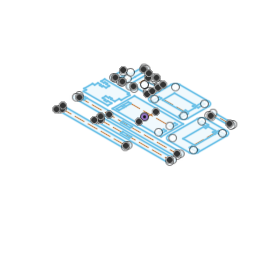
laser cut parts v7 (Autodesk Fusion 360 design; units mm, degrees)
Autodesk Fusion 360 part; units mm, degrees
note: some values were not read from the file. Set by a fixed rule: which sketch regions a step uses.
sketch "Sketch1" plane through (0, 0, 0) normal (0, 0, 1) x (1, 0, 0)
  line L0 (-61.9661, -10.0098) -> (-33.3218, -10.0098)
  line L1 (-33.3218, 14.9902) -> (-61.9661, 14.9902)
  line L2 (-33.3218, 13.3981) -> (-30.7818, 13.3981)
  line L3 (-30.7818, 13.3981) -> (-30.7818, 3.3981)
  line L4 (-30.7818, 3.3981) -> (-33.3218, 3.3981)
  line L5 (-61.9661, 3.271) -> (-64.5061, 3.271)
  line L6 (-64.5061, 3.271) -> (-64.5061, -6.729)
  line L7 (-64.5061, -6.729) -> (-61.9661, -6.729)
  line L8 (-58.6214, 11.9525) -> (-55.9714, 11.9525)
  line L9 (-55.9714, 5.9525) -> (-58.6214, 5.9525)
  line L10 (-58.6214, 10.8025) -> (-61.9661, 10.8025)
  line L11 (-58.6214, 7.1025) -> (-61.9661, 7.1025)
  line L12 (-58.6214, 5.9525) -> (-58.6214, 7.1025)
  line L13 (-58.6214, 10.8025) -> (-58.6214, 11.9525)
  line L14 (-61.9661, 14.9902) -> (-61.9661, 10.8025)
  line L15 (-61.9661, 7.1025) -> (-61.9661, 3.271)
  line L16 (-61.9661, -6.729) -> (-61.9661, -10.0098)
  line L17 (-33.3218, 13.3981) -> (-33.3218, 14.9902)
  line L18 (-55.9714, 10.8025) -> (-52.3522, 10.8025)
  line L19 (-55.9714, 7.1025) -> (-52.3522, 7.1025)
  line L20 (-52.3522, 7.1025) -> (-52.3522, 10.8025)
  line L21 (-55.9714, 11.9525) -> (-55.9714, 10.8025)
  line L22 (-55.9714, 7.1025) -> (-55.9714, 5.9525)
  line L23 (-40.6135, -1.7451) -> (-43.9582, -1.7451)
  line L24 (-40.6135, -1.7451) -> (-40.6135, -0.5951)
  line L25 (-40.6135, -0.5951) -> (-37.9635, -0.5951)
  line L26 (-37.9635, -0.5951) -> (-37.9635, -1.7451)
  line L27 (-37.9635, -5.4451) -> (-37.9635, -6.5951)
  line L28 (-37.9635, -6.5951) -> (-40.6135, -6.5951)
  line L29 (-40.6135, -6.5951) -> (-40.6135, -5.4451)
  line L30 (-40.6135, -5.4451) -> (-43.9582, -5.4451)
  line L31 (-43.9582, -1.7451) -> (-43.9582, -5.4451)
  line L32 (-37.9635, -1.7451) -> (-33.3218, -1.7451)
  line L33 (-37.9635, -5.4451) -> (-33.3218, -5.4451)
  line L34 (-33.3218, -10.0098) -> (-33.3218, -5.4451)
  line L35 (-33.3218, -1.7451) -> (-33.3218, 3.3981)
  dimension "d35" = 10
  dimension "d36" = 2.54
  dimension "d37" = 2.54
  dimension "d39" = 6
  dimension "d40" = 2.65
  dimension "d43" = 6
  dimension "d44" = 2.65
  dimension "d113" = 28.6443
  dimension "d114" = 10
  constraint horizontal L0
  constraint vertical L34
  constraint horizontal L1
  constraint vertical L14
  constraint horizontal L2
  constraint vertical L3
  constraint horizontal L4
  constraint coincident L2.start L34
  constraint horizontal L5
  constraint vertical L6
  constraint horizontal L7
  constraint coincident L5.start L14
  constraint horizontal L8
  constraint vertical L21
  constraint horizontal L9
  constraint vertical L12
  constraint perpendicular L10 L14
  constraint coincident L11.end L14
  constraint perpendicular L11 L14
  constraint collinear L12 L13
  constraint collinear L14 L15
  constraint collinear L15 L16
  constraint collinear L17 L34
  constraint perpendicular L18 L21
  constraint coincident L19.start L21
  constraint perpendicular L19 L21
  constraint perpendicular L18 L20
  constraint collinear L21 L22
  constraint horizontal L25
  constraint vertical L26
  constraint horizontal L28
  constraint vertical L29
  constraint collinear L24 L29
  constraint coincident L27.start L26
  constraint collinear L26 L27
  constraint perpendicular L30 L31
  constraint coincident L32.end L34
  constraint perpendicular L32 L34
  constraint perpendicular L33 L34
  constraint collinear L34 L35
  measures "d35" distance of L2.end L3.end
  measures "d36" distance of L2.start L2.end
  measures "d37" distance of L5.start L5.end
  measures "d39" distance of L8.start L9.end
  measures "d40" distance of L8.start L8.end
  measures "d43" distance of L24.end L28.end
  measures "d44" distance of L24.end L25.end
  measures "d113" distance of L1.start L1.end
  measures "d114" distance of L5.end L6.end
sketch "Sketch2" plane through (0, 0, 0) normal (0, 0, 1) x (1, 0, 0)
  line L0 (-27.3063, 15.4747) -> (30.0656, 15.4747)
  line L1 (30.0656, 15.4747) -> (30.0656, -10.5253)
  line L2 (30.0656, -10.5253) -> (-27.3063, -10.5253)
  line L3 (-27.3063, -10.5253) -> (-27.3063, 15.4747)
  line L4 (-21.7678, 5.5369) -> (24.2322, 5.5369) construction
  line L5 (-21.7678, 5.5369) -> (-24.6678, 5.5369)
  line L6 (-24.6678, 5.5369) -> (-24.6678, -0.4631)
  line L7 (-24.6678, -0.4631) -> (-21.7678, -0.4631)
  line L8 (-21.7678, -0.4631) -> (-21.7678, 5.5369)
  line L9 (-21.7678, -2.4631) -> (-24.6678, -2.4631)
  line L10 (-24.6678, -2.4631) -> (-24.6678, -8.4631)
  line L11 (-24.6678, -8.4631) -> (-21.7678, -8.4631)
  line L12 (-21.7678, -8.4631) -> (-21.7678, -2.4631)
  line L13 (24.0392, 11.4747) -> (24.0392, 5.4747)
  line L14 (26.9392, 11.4747) -> (24.0392, 11.4747)
  line L15 (26.9392, 5.4747) -> (26.9392, 11.4747)
  line L16 (24.0392, 5.4747) -> (26.9392, 5.4747)
  line L17 (26.9392, -1.5253) -> (24.0392, -1.5253)
  line L18 (24.0392, -7.5253) -> (26.9392, -7.5253)
  line L19 (26.9392, -7.5253) -> (26.9392, -1.5253)
  line L20 (24.0392, -1.5253) -> (24.0392, -7.5253)
  line L21 (1.5442, 11.8441) -> (1.5442, -8.1559) construction
  circle A0 centre (1.5442, 11.8441) radius 0.85
  circle A1 centre (1.5442, -8.1559) radius 0.8502
  line L22 (-49.0766, 46.3412) -> (-49.0766, 47.8412) construction
  circle A2 centre (-49.0766, 47.8412) radius 1.5
  line L23 (-49.0766, 46.3412) -> (-49.0766, 51.2139) construction
  line L24 (-49.0766, 51.2139) -> (-50.2257, 51.2139)
  line L25 (-51.7257, 49.7139) -> (-51.7257, 37.2072)
  line L26 (-49.0766, 51.2139) -> (-49.0766, 46.3412) construction
  line L27 (-46.3309, 35.2072) -> (-46.3309, 49.7139)
  line L28 (-47.8309, 51.2139) -> (-49.0766, 51.2139)
  line L29 (-46.3309, 35.2072) -> (-46.3309, 21.8412)
  line L30 (-48.3309, 19.8412) -> (-50.3309, 19.8412)
  line L31 (-52.3309, 21.8412) -> (-52.3309, 28.5115)
  line L32 (-64.4221, -95.7993) -> (-64.4221, -95.7993)
  line L33 (-54.3309, 35.2072) -> (-53.7257, 35.2072)
  line L34 (-54.3309, 35.2072) -> (-58.3309, 35.2072)
  line L35 (-60.3309, 33.2072) -> (-60.3309, 21.8412)
  line L36 (-54.3309, 28.5115) -> (-54.3309, 21.8412)
  line L37 (-56.3309, 19.8412) -> (-58.3309, 19.8412)
  line L38 (-49.0766, 28.8412) -> (-49.0766, 23.0481) construction
  circle A3 centre (-49.0766, 23.0481) radius 1.5
  circle A4 centre (-57.3309, 23.0481) radius 1.5
  arc A5 (-60.3309, 21.8412) -> (-58.3309, 19.8412) centre (-58.3309, 21.8412) ccw
  arc A6 (-56.3309, 19.8412) -> (-54.3309, 21.8412) centre (-56.3309, 21.8412) ccw
  arc A7 (-58.3309, 35.2072) -> (-60.3309, 33.2072) centre (-58.3309, 33.2072) ccw
  arc A8 (-52.3309, 21.8412) -> (-50.3309, 19.8412) centre (-50.3309, 21.8412) ccw
  arc A9 (-48.3309, 19.8412) -> (-46.3309, 21.8412) centre (-48.3309, 21.8412) ccw
  arc A10 (-53.7257, 35.2072) -> (-51.7257, 37.2072) centre (-53.7257, 37.2072) ccw
  arc A11 (-50.2257, 51.2139) -> (-51.7257, 49.7139) centre (-50.2257, 49.7139) ccw
  arc A12 (-46.3309, 49.7139) -> (-47.8309, 51.2139) centre (-47.8309, 49.7139) ccw
  line L39 (-37.6449, 41.9803) -> (-37.6449, 24.6803) construction
  circle A13 centre (-37.6449, 41.9803) radius 1.5
  circle A14 centre (-37.6449, 24.6803) radius 1.5
  line L40 (-39.9332, 46.9834) -> (-34.8949, 46.9834)
  line L41 (-34.8949, 20.5727) -> (-39.9332, 20.5727)
  line L42 (-41.9332, 22.5727) -> (-41.9332, 44.9834)
  line L43 (-37.6449, 41.9803) -> (-32.8949, 41.9803) construction
  line L44 (-21.7527, 26.8103) -> (-21.7527, 28.8103)
  line L45 (-23.7527, 30.8103) -> (-32.8949, 30.8103)
  line L46 (-32.8949, 32.8103) -> (-32.8949, 32.9834) construction
  line L47 (-32.8949, 37.8103) -> (-23.8949, 37.8103)
  line L48 (-21.8949, 39.8103) -> (-21.8949, 41.8103)
  line L49 (-23.8949, 43.8103) -> (-32.8949, 43.8103)
  line L50 (-32.8949, 44.9834) -> (-32.8949, 43.8103)
  line L51 (-32.8949, 37.8103) -> (-32.8949, 30.8103)
  line L52 (-32.8949, 24.8103) -> (-32.8949, 22.5727)
  line L53 (-32.8949, 24.8103) -> (-23.7527, 24.8103)
  circle A15 centre (-24.5988, 40.8103) radius 1.5
  circle A16 centre (-24.5988, 27.5507) radius 1.5
  line L54 (-49.0766, 23.0481) -> (-57.3309, 23.0481) construction
  line L55 (-32.8949, 43.8103) -> (-30.3549, 43.8103) construction
  arc A17 (-39.9332, 46.9834) -> (-41.9332, 44.9834) centre (-39.9332, 44.9834) ccw
  arc A18 (-32.8949, 44.9834) -> (-34.8949, 46.9834) centre (-34.8949, 44.9834) ccw
  arc A19 (-41.9332, 22.5727) -> (-39.9332, 20.5727) centre (-39.9332, 22.5727) ccw
  arc A20 (-34.8949, 20.5727) -> (-32.8949, 22.5727) centre (-34.8949, 22.5727) ccw
  arc A21 (-23.7527, 24.8103) -> (-21.7527, 26.8103) centre (-23.7527, 26.8103) ccw
  arc A22 (-21.7527, 28.8103) -> (-23.7527, 30.8103) centre (-23.7527, 28.8103) ccw
  arc A23 (-23.8949, 37.8103) -> (-21.8949, 39.8103) centre (-23.8949, 39.8103) ccw
  arc A24 (-21.8949, 41.8103) -> (-23.8949, 43.8103) centre (-23.8949, 41.8103) ccw
  line L56 (-53.3309, 29.5115) -> (-54.3309, 29.5115)
  line L57 (-54.3309, 29.5115) -> (-54.3309, 28.5115)
  line L58 (-52.3309, 28.5115) -> (-52.3309, 29.5046)
  line L59 (-52.3309, 29.5046) -> (-53.3309, 29.5115)
  line L60 (17.4575, 27.8424) -> (-6.5425, 27.8424)
  line L61 (-6.5425, 27.8424) -> (-6.5425, 41.8424)
  line L62 (-6.5425, 41.8424) -> (17.4575, 41.8424)
  line L63 (27.0896, 48.5722) -> (27.0896, 24.0668)
  line L64 (22.0896, 19.0668) -> (-12.121, 19.0668)
  line L65 (-17.121, 24.0668) -> (-17.121, 48.5722)
  line L66 (-12.121, 53.5722) -> (22.0896, 53.5722)
  line L67 (19.389, 28.8858) -> (-8.997, 28.8858) construction
  line L68 (-8.997, 28.8858) -> (-11.897, 28.8858)
  line L69 (-11.897, 28.8858) -> (-11.897, 21.2858)
  line L70 (-11.897, 21.2858) -> (-8.997, 21.2858)
  line L71 (-8.997, 21.2858) -> (-8.997, 28.8858)
  line L72 (19.389, 28.8858) -> (19.389, 21.2858)
  line L73 (22.289, 28.8858) -> (19.389, 28.8858)
  line L74 (19.389, 21.2858) -> (22.289, 21.2858)
  line L75 (22.289, 21.2858) -> (22.289, 28.8858)
  line L76 (17.4575, 30.8424) -> (20.5266, 30.8424)
  line L77 (20.5266, 30.8424) -> (20.5266, 39.3145)
  line L78 (20.5266, 39.3145) -> (17.4575, 39.3145)
  line L79 (17.4575, 41.8424) -> (17.4575, 39.3145)
  line L80 (17.4575, 30.8424) -> (17.4575, 27.8424)
  line L81 (56.9333, 43.0759) -> (37.9333, 43.0759) construction
  line L82 (37.9333, 43.0759) -> (37.9333, 40.0759) construction
  circle A25 centre (56.9333, 43.0759) radius 1.5
  circle A26 centre (37.9333, 40.0759) radius 1.5
  line L83 (40.5113, 45.3188) -> (59.9333, 45.3188)
  line L84 (60.9333, 44.3188) -> (60.9333, 42.0759)
  line L85 (59.9333, 41.0759) -> (40.5113, 41.0759)
  line L86 (35.4581, 39.0759) -> (35.4581, 44.3188)
  line L87 (36.4581, 45.3188) -> (40.5113, 45.3188)
  line L88 (39.5113, 38.0759) -> (36.4581, 38.0759)
  line L89 (40.5113, 41.0759) -> (40.5113, 39.0759)
  arc A27 (36.4581, 45.3188) -> (35.4581, 44.3188) centre (36.4581, 44.3188) ccw
  arc A28 (35.4581, 39.0759) -> (36.4581, 38.0759) centre (36.4581, 39.0759) ccw
  arc A29 (39.5113, 38.0759) -> (40.5113, 39.0759) centre (39.5113, 39.0759) ccw
  arc A30 (60.9333, 44.3188) -> (59.9333, 45.3188) centre (59.9333, 44.3188) ccw
  arc A31 (59.9333, 41.0759) -> (60.9333, 42.0759) centre (59.9333, 42.0759) ccw
  arc A32 (27.0896, 48.5722) -> (22.0896, 53.5722) centre (22.0896, 48.5722) ccw
  arc A33 (22.0896, 19.0668) -> (27.0896, 24.0668) centre (22.0896, 24.0668) ccw
  arc A34 (-17.121, 24.0668) -> (-12.121, 19.0668) centre (-12.121, 24.0668) ccw
  arc A35 (-12.121, 53.5722) -> (-17.121, 48.5722) centre (-12.121, 48.5722) ccw
  line L90 (22.289, 40.9858) -> (22.289, 48.5858)
  line L91 (19.389, 40.9858) -> (22.289, 40.9858)
  line L92 (19.389, 48.5858) -> (19.389, 40.9858)
  line L93 (22.289, 48.5858) -> (19.389, 48.5858)
  line L94 (47.4987, 27.5806) -> (47.4987, 24.5115)
  line L95 (57.9274, 29.343) -> (57.9274, 26.443)
  line L96 (55.9708, 24.5115) -> (58.9708, 24.5115)
  line L97 (67.7464, 29.1436) -> (67.7464, -5.067)
  line L98 (57.9274, 26.443) -> (65.5274, 26.443)
  line L99 (62.7464, -10.067) -> (38.241, -10.067)
  line L100 (57.9274, 26.443) -> (57.9274, -1.943) construction
  arc A36 (67.7464, 29.1436) -> (62.7464, 34.1436) centre (62.7464, 29.1436) ccw
  line L101 (65.5274, -4.843) -> (65.5274, -1.943)
  line L102 (57.9274, -4.843) -> (65.5274, -4.843)
  arc A37 (62.7464, -10.067) -> (67.7464, -5.067) centre (62.7464, -5.067) ccw
  line L103 (57.9274, -1.943) -> (57.9274, -4.843)
  line L104 (38.2274, 26.443) -> (45.8274, 26.443)
  line L105 (58.9708, 0.5115) -> (44.9708, 0.5115)
  line L106 (65.5274, 26.443) -> (65.5274, 29.343)
  line L107 (58.9708, 24.5115) -> (58.9708, 0.5115)
  line L108 (65.5274, -1.943) -> (57.9274, -1.943)
  line L109 (55.9708, 27.5806) -> (47.4987, 27.5806)
  line L110 (65.5274, 29.343) -> (57.9274, 29.343)
  line L111 (38.2274, 29.343) -> (38.2274, 26.443)
  line L112 (44.9708, 0.5115) -> (44.9708, 24.5115)
  arc A38 (33.241, -5.067) -> (38.241, -10.067) centre (38.241, -5.067) ccw
  line L113 (45.8274, 29.343) -> (38.2274, 29.343)
  line L114 (33.241, -5.067) -> (33.241, 29.1436)
  line L115 (45.8274, 26.443) -> (45.8274, 29.343)
  line L116 (55.9708, 24.5115) -> (55.9708, 27.5806)
  arc A39 (38.241, 34.1436) -> (33.241, 29.1436) centre (38.241, 29.1436) ccw
  line L117 (38.241, 34.1436) -> (62.7464, 34.1436)
  line L118 (44.9708, 24.5115) -> (47.4987, 24.5115)
  line L119 (-58.2128, -18.4866) -> (56.7872, -18.4866) construction
  circle A40 centre (-58.2128, -18.4866) radius 1.5
  circle A41 centre (56.7872, -18.4866) radius 1.5
  circle A42 centre (-23.2128, -18.4866) radius 1.5
  line L120 (60.7197, -16.6366) -> (60.7197, -20.3366)
  line L121 (58.8197, -22.2366) -> (-60.2829, -22.2366)
  line L122 (-62.1829, -20.3366) -> (-62.1829, -16.6366)
  arc A43 (-60.2829, -14.7366) -> (-62.1829, -16.6366) centre (-60.2829, -16.6366) ccw
  arc A44 (-62.1829, -20.3366) -> (-60.2829, -22.2366) centre (-60.2829, -20.3366) ccw
  arc A45 (60.7197, -16.6366) -> (58.8197, -14.7366) centre (58.8197, -16.6366) ccw
  arc A46 (58.8197, -22.2366) -> (60.7197, -20.3366) centre (58.8197, -20.3366) ccw
  line L123 (-22.8073, -29.1187) -> (58.7927, -29.1187) construction
  circle A47 centre (-22.8073, -29.1187) radius 1.5
  circle A48 centre (58.7927, -29.1187) radius 1.5
  line L124 (-24.3346, -25.3687) -> (60.5465, -25.3687)
  line L125 (62.5465, -27.3687) -> (62.5465, -30.8687)
  line L126 (60.5465, -32.8687) -> (-24.3346, -32.8687)
  line L127 (-26.3346, -30.8687) -> (-26.3346, -27.3687)
  arc A49 (-24.3346, -25.3687) -> (-26.3346, -27.3687) centre (-24.3346, -27.3687) ccw
  arc A50 (-26.3346, -30.8687) -> (-24.3346, -32.8687) centre (-24.3346, -30.8687) ccw
  arc A51 (62.5465, -27.3687) -> (60.5465, -25.3687) centre (60.5465, -27.3687) ccw
  arc A52 (60.5465, -32.8687) -> (62.5465, -30.8687) centre (60.5465, -30.8687) ccw
  line L128 (-56.5917, -40.3853) -> (18.4083, -40.3853) construction
  circle A53 centre (-56.5917, -40.3853) radius 1.5
  circle A54 centre (18.4083, -40.3853) radius 1.5
  line L129 (-57.5917, -36.6353) -> (19.4083, -36.6353)
  line L130 (21.4083, -38.6353) -> (21.4083, -42.1353)
  line L131 (19.4083, -44.1353) -> (-57.5917, -44.1353)
  line L132 (-59.5917, -42.1353) -> (-59.5917, -38.6353)
  arc A55 (21.4083, -38.6353) -> (19.4083, -36.6353) centre (19.4083, -38.6353) ccw
  arc A56 (19.4083, -44.1353) -> (21.4083, -42.1353) centre (19.4083, -42.1353) ccw
  arc A57 (-57.5917, -36.6353) -> (-59.5917, -38.6353) centre (-57.5917, -38.6353) ccw
  arc A58 (-59.5917, -42.1353) -> (-57.5917, -44.1353) centre (-57.5917, -42.1353) ccw
  line L133 (-8.1006, -17.2066) -> (2.4677, -17.2066)
  line L134 (2.4677, -17.2066) -> (2.4677, -19.7466)
  line L135 (2.4677, -19.7466) -> (-8.1006, -19.7466)
  line L136 (-8.1006, -19.7466) -> (-8.1006, -17.2066)
  line L137 (2.4677, -28.0285) -> (12.4677, -28.0285)
  line L138 (12.4677, -28.0285) -> (12.4677, -30.5685)
  line L139 (12.4677, -30.5685) -> (2.4677, -30.5685)
  line L140 (2.4677, -30.5685) -> (2.4677, -28.0285)
  line L141 (-53.0976, -14.7366) -> (-53.0976, -18.4866)
  line L142 (-53.0976, -18.4866) -> (-54.8276, -18.4866)
  line L143 (-54.8276, -18.4866) -> (-54.8276, -14.7366)
  line L144 (-60.2829, -14.7366) -> (-54.8276, -14.7366)
  line L145 (-53.0976, -14.7366) -> (58.8197, -14.7366)
  point P0 (24.0522, -7.4631)
  point P1 (-60.3309, 35.2072)
  point P2 (-41.9332, 46.9834)
  point P3 (-32.8949, 46.9834)
  point P4 (-21.7527, 24.8103)
  point P5 (-21.7527, 30.8103)
  point P6 (-21.8949, 37.8103)
  point P7 (-21.8949, 43.8103)
  point P8 (-26.3346, -25.3687)
  point P9 (-26.3346, -32.8687)
  point P10 (-59.5917, -36.6353)
  point P11 (-59.5917, -44.1353)
  dimension "d335" = 2.54
  dimension "d336" = 2.54
  dimension "d337" = 3.81
  dimension "d338" = 23
  dimension "d341" = 10.0076
  dimension "d342" = 10.0076
  dimension "d46" = 46
  dimension "d47" = 6
  dimension "d48" = 2.9
  dimension "d50" = 2.9
  dimension "d51" = 6
  dimension "d52" = 26
  dimension "d53" = 6
  dimension "d54" = 2.9
  dimension "d55" = 2
  dimension "d56" = 6
  dimension "d57" = 2.9
  dimension "d58" = 20
  dimension "d59" = 1.7
  dimension "d61" = 3
  dimension "d64" = 6
  dimension "d66" = 9
  dimension "d68" = 3
  dimension "d69" = 3
  dimension "d70" = 3
  dimension "d71" = 2
  dimension "d73" = 1.5
  dimension "d74" = 17.3
  dimension "d75" = 3
  dimension "d76" = 3
  dimension "d78" = 7
  dimension "d79" = 4
  dimension "d80" = 9.9378
  dimension "d81" = 2.7457
  dimension "d82" = 6
  dimension "d83" = 7
  dimension "d85" = 6
  dimension "d86" = 3
  dimension "d87" = 3
  dimension "d90" = 4.2883
  dimension "d92" = 2
  dimension "d93" = 24
  dimension "d95" = 28.386
  dimension "d96" = 7.6
  dimension "d97" = 2.9
  dimension "d98" = 7.6
  dimension "d99" = 2.9
  dimension "d101" = 3
  dimension "d102" = 3
  dimension "d103" = 3
  dimension "d104" = 2
  dimension "d105" = 1
  dimension "d115" = 5
  dimension "d116" = 7.6
  dimension "d117" = 2.9
  dimension "d118" = 12.1
  dimension "d119" = 24
  dimension "d120" = 28.386
  dimension "d121" = 7.6
  dimension "d122" = 2.9
  dimension "d123" = 7.6
  dimension "d124" = 2.9
  dimension "d125" = 5
  dimension "d126" = 7.6
  dimension "d127" = 2.9
  dimension "d128" = 12.1
  dimension "d136" = 115
  dimension "d137" = 3
  dimension "d138" = 3
  dimension "d139" = 3
  dimension "d140" = 35
  dimension "d141" = 7.5
  dimension "d142" = 3.75
  dimension "d143" = 1.9
  dimension "d144" = 81.6
  dimension "d145" = 3
  dimension "d146" = 3
  dimension "d147" = 7.5
  dimension "d148" = 3.75
  dimension "d149" = 2
  dimension "d150" = 75
  dimension "d151" = 3
  dimension "d152" = 3
  dimension "d153" = 7.5
  dimension "d154" = 3.75
  dimension "d155" = 2
  dimension "d156" = 2.54
  dimension "d157" = 2.47
  dimension "d158" = 2.54
  dimension "d159" = 2.6598
  dimension "d162" = 1.73
  constraint horizontal L0
  constraint vertical L1
  constraint horizontal L2
  constraint vertical L3
  constraint horizontal L4
  constraint horizontal L5
  constraint vertical L6
  constraint horizontal L7
  constraint vertical L8
  constraint horizontal L9
  constraint vertical L10
  constraint horizontal L11
  constraint vertical L12
  constraint collinear L8 L12
  constraint horizontal L14
  constraint vertical L13
  constraint horizontal L16
  constraint vertical L15
  constraint horizontal L17
  constraint vertical L20
  constraint horizontal L18
  constraint vertical L19
  constraint perpendicular L4 L21
  constraint coincident L21.start A0.centre
  constraint coincident L21.end A1.centre
  constraint coincident L22.end A2.centre
  constraint coincident A2 L22.start
  constraint perpendicular L34 L35
  constraint perpendicular L35 L37
  constraint coincident L38.end A3.centre
  constraint collinear L30 L37
  constraint tangent L35 A5
  constraint tangent L37 A5
  constraint tangent L36 A6
  constraint tangent L37 A6
  constraint equal A5 A6
  constraint coincident P1 L34
  constraint coincident P1 L35
  constraint tangent L34 A7
  constraint tangent L35 A7
  constraint equal A5 A7
  constraint tangent L30 A8
  constraint tangent L31 A8
  constraint equal A5 A8
  constraint tangent L29 A9
  constraint tangent L30 A9
  constraint equal A5 A9
  constraint tangent L25 A10
  constraint equal A5 A10
  constraint tangent L24 A11
  constraint tangent L25 A11
  constraint tangent L27 A12
  constraint tangent L28 A12
  constraint equal A11 A12
  constraint vertical L39
  constraint coincident L39.start A13.centre
  constraint coincident L39.end A14.centre
  constraint horizontal L40
  constraint vertical L50
  constraint horizontal L41
  constraint vertical L42
  constraint perpendicular L39 L43
  constraint coincident L45.end L50
  constraint perpendicular L45 L50
  constraint perpendicular L45 L46
  constraint perpendicular L46 L47
  constraint perpendicular L47 L48
  constraint perpendicular L48 L49
  constraint collinear L50 L51
  constraint collinear L51 L52
  constraint perpendicular L36 L54
  constraint coincident A4.centre L54.end
  constraint perpendicular L50 L55
  constraint coincident P2 L40
  constraint coincident P2 L42
  constraint tangent L40 A17
  constraint tangent L42 A17
  constraint coincident P3 L40
  constraint coincident P3 L50
  constraint tangent L40 A18
  constraint tangent L50 A18
  constraint equal A17 A18
  constraint tangent L41 A19
  constraint tangent L42 A19
  constraint equal A17 A19
  constraint tangent L41 A20
  constraint tangent L52 A20
  constraint equal A17 A20
  constraint coincident P4 L44
  constraint coincident P4 L53
  constraint tangent L44 A21
  constraint tangent L53 A21
  constraint equal A17 A21
  constraint coincident P5 L44
  constraint coincident P5 L45
  constraint tangent L44 A22
  constraint tangent L45 A22
  constraint equal A17 A22
  constraint coincident L51.start L47
  constraint coincident L51.end L45
  constraint coincident L45.end L46
  constraint coincident P6 L47
  constraint coincident P6 L48
  constraint tangent L47 A23
  constraint tangent L48 A23
  constraint equal A17 A23
  constraint coincident P7 L48
  constraint coincident P7 L49
  constraint tangent L48 A24
  constraint tangent L49 A24
  constraint equal A17 A24
  constraint horizontal L53
  constraint perpendicular L36 L56
  constraint perpendicular L56 L57
  constraint parallel L31 L58
  constraint perpendicular L72 L73
  constraint perpendicular L72 L74
  constraint perpendicular L74 L75
  constraint collinear L79 L80
  constraint perpendicular L81 L82
  constraint coincident L81.start A25.centre
  constraint coincident L82.end A26.centre
  constraint coincident L85 L89.start
  constraint collinear L83 L87
  constraint tangent L86 A27
  constraint tangent L87 A27
  constraint tangent L86 A28
  constraint tangent L88 A28
  constraint equal A27 A28
  constraint tangent L88 A29
  constraint tangent L89 A29
  constraint equal A27 A29
  constraint tangent L83 A30
  constraint tangent L84 A30
  constraint equal A27 A30
  constraint tangent L84 A31
  constraint tangent L85 A31
  constraint equal A27 A31
  constraint tangent L63 A32
  constraint tangent L66 A32
  constraint tangent L63 A33
  constraint tangent L64 A33
  constraint equal A32 A33
  constraint tangent L64 A34
  constraint tangent L65 A34
  constraint equal A32 A34
  constraint tangent L65 A35
  constraint tangent L66 A35
  constraint equal A32 A35
  constraint perpendicular L92 L93
  constraint perpendicular L91 L92
  constraint perpendicular L90 L91
  constraint horizontal L118
  constraint vertical L107
  constraint horizontal L105
  constraint vertical L112
  constraint horizontal L117
  constraint vertical L97
  constraint horizontal L99
  constraint vertical L114
  constraint perpendicular L95 L98
  constraint perpendicular L98 L106
  constraint perpendicular L106 L110
  constraint vertical L116
  constraint horizontal L109
  constraint vertical L94
  constraint collinear L96 L118
  constraint tangent A39 L117
  constraint tangent L114 A39
  constraint tangent A36 L117
  constraint tangent L97 A36
  constraint equal A36 A39
  constraint tangent L97 A37
  constraint tangent L99 A37
  constraint equal A37 A39
  constraint tangent L99 A38
  constraint tangent A38 L114
  constraint equal A38 A39
  constraint perpendicular L104 L111
  constraint perpendicular L104 L115
  constraint perpendicular L113 L115
  constraint horizontal L119
  constraint coincident L119.start A40.centre
  constraint coincident L119.end A41.centre
  constraint coincident L119 A42.centre
  constraint horizontal L144
  constraint vertical L120
  constraint horizontal L121
  constraint vertical L122
  constraint tangent A43 L144
  constraint tangent L122 A43
  constraint tangent L121 A44
  constraint tangent L122 A44
  constraint equal A43 A44
  constraint tangent A45 L144
  constraint tangent L120 A45
  constraint equal A43 A45
  constraint tangent L120 A46
  constraint tangent L121 A46
  constraint equal A43 A46
  constraint parallel L121 L123
  constraint coincident L123.start A47.centre
  constraint coincident L123.end A48.centre
  constraint horizontal L124
  constraint vertical L125
  constraint horizontal L126
  constraint vertical L127
  constraint coincident P8 L124
  constraint coincident P8 L127
  constraint tangent L124 A49
  constraint tangent L127 A49
  constraint coincident P9 L126
  constraint coincident P9 L127
  constraint tangent L126 A50
  constraint tangent L127 A50
  constraint equal A49 A50
  constraint tangent L124 A51
  constraint tangent L125 A51
  constraint equal A49 A51
  constraint tangent L125 A52
  constraint tangent L126 A52
  constraint equal A49 A52
  constraint parallel L119 L128
  constraint coincident L128.start A53.centre
  constraint coincident L128.end A54.centre
  constraint horizontal L129
  constraint vertical L130
  constraint horizontal L131
  constraint vertical L132
  constraint tangent L129 A55
  constraint tangent L130 A55
  constraint tangent L130 A56
  constraint tangent L131 A56
  constraint equal A55 A56
  constraint coincident P10 L129
  constraint coincident P10 L132
  constraint tangent L129 A57
  constraint tangent L132 A57
  constraint equal A55 A57
  constraint coincident P11 L131
  constraint coincident P11 L132
  constraint tangent L131 A58
  constraint tangent L132 A58
  constraint equal A55 A58
  constraint horizontal L133
  constraint vertical L134
  constraint horizontal L135
  constraint vertical L136
  constraint horizontal L137
  constraint vertical L138
  constraint horizontal L139
  constraint vertical L140
  constraint collinear L134 L140
  constraint vertical L141
  constraint horizontal L142
  constraint vertical L143
  constraint coincident L119 L141.end
  constraint collinear L144 L145
  measures "d46" distance of L4.start L4.end
  measures "d47" distance of L4.start L7.end
  measures "d48" distance of L4.start L5.end
  measures "d50" distance of L10.end L11.end
  measures "d51" distance of L9.end L10.end
  measures "d52" distance of L0.end L1.end
  measures "d53" distance of L15.start L14.start
  measures "d54" distance of L13.start L14.start
  measures "d55" distance of L7 L9
  measures "d56" distance of L18.end L17.start
  measures "d57" distance of L17.end L17.start
  measures "d58" distance of L21.start L21.end
  measures "d59" diameter of A0
  measures "d61" diameter of A2
  measures "d64" distance of L33.start P1
  measures "d66" distance of L30 L38.start
  measures "d68" diameter of A3
  measures "d69" diameter of A4
  measures "d70" distance of L35 A4.centre
  measures "d71" radius of A5
  measures "d73" radius of A11
  measures "d74" distance of L39.start L39.end
  measures "d75" diameter of A13
  measures "d76" diameter of A14
  measures "d78" distance of L16 L17
  measures "d79" distance of L0 L14
  measures "d80" distance of L0 L5
  measures "d81" distance of L29 L38.end
  measures "d82" distance of P4 P5
  measures "d83" distance of L45.end L47.start
  measures "d85" distance of P6 P7
  measures "d86" diameter of A15
  measures "d87" diameter of A16
  measures "d90" distance of L39.start L42
  measures "d92" radius of A17
  measures "d93" distance of L62.end L61.end
  measures "d95" distance of L67.start L67.end
  measures "d96" distance of L67.end L70.end
  measures "d97" distance of L67.end L68.end
  measures "d98" distance of L74.end L73.start
  measures "d99" distance of L67.start L73.start
  measures "d101" distance of L81.end L82.end
  measures "d102" diameter of A25
  measures "d103" diameter of A26
  measures "d104" distance of L81.start L85
  measures "d105" radius of A27
  measures "d115" radius of A32
  measures "d116" distance of L90.end L90.start
  measures "d117" distance of L90.end L92.start
  measures "d118" distance of L73 L91
  measures "d119" distance of L105.end L112.end
  measures "d120" distance of L95.end L100.end
  measures "d121" distance of L101.end L100.end
  measures "d122" distance of L102.start L100.end
  measures "d123" distance of L95.start L106.end
  measures "d124" distance of L95.start L95.end
  measures "d125" radius of A39
  measures "d126" distance of L111.start L113.start
  measures "d127" distance of L111.start L104.start
  measures "d128" distance of L95 L115
  measures "d136" distance of L119.start L119.end
  measures "d137" diameter of A40
  measures "d138" diameter of A41
  measures "d139" diameter of A42
  measures "d140" distance of L119.start A42.centre
  measures "d141" distance of L121 L144
  measures "d142" distance of L119.end L144
  measures "d143" radius of A43
  measures "d144" distance of L123.start L123.end
  measures "d145" diameter of A47
  measures "d146" diameter of A48
  measures "d147" distance of P8 P9
  measures "d148" distance of L123.end L124
  measures "d149" radius of A49
  measures "d150" distance of L128.start L128.end
  measures "d151" diameter of A53
  measures "d152" diameter of A54
  measures "d153" distance of P10 P11
  measures "d154" distance of L128 L129
  measures "d155" radius of A55
  measures "d156" distance of L133.end L134.end
  measures "d157" distance of L133 L144
  measures "d158" distance of L137.start L139.end
  measures "d159" distance of L124 L137
  measures "d162" distance of L141 L143
extrude "Extrude2" add sketch "Sketch2" along normal blind 2.54 contours L24 L25 L27 L28 L29 L30 L31 L33 L34 L35 L36 L37 A5 A6 A7 A8 A9 A10 A11 A12 L56 L57 L58 L59 makes body 1
extrude "Extrude1" add sketch "Sketch2" along normal blind 2.54 separate body contours L63 L64 L65 L66 A32 A33 A34 A35 | L97 L99 A36 A37 A38 L114 A39 L117 makes body 2 at (0.2419, 48.0001, 0) makes body 3 at (38.8131, 7.2959, 0)
extrude "Extrude3" add sketch "Sketch2" along normal blind 2.54 separate body contours L40 L41 L42 L44 L45 L47 L48 L49 L50 L51 L52 L53 A17 A18 A19 A20 A21 A22 A23 A24 makes body 4
extrude "Extrude4" add sketch "Sketch2" along normal blind 2.54 separate body contours L120 L121 L122 A43 A44 A45 A46 L141 L142 L143 L144 L145 | L124 L125 L126 L127 A49 A50 A51 A52 | L129 L130 L131 L132 A55 A56 A57 A58 makes body 5 at (-43.6344, -17.1964, 0) makes body 6 at (12.8932, -26.2553, 0) makes body 7 at (-6.9582, -37.5452, 0)
